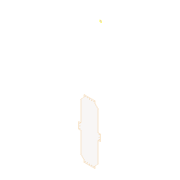
# Autodesk Inventor part: Test_Swerve_Center
Saved by Autodesk Inventor 2021 (Build 250183000, 183)
## iProperties
Created: 2023-03-29
Part Number: Test_Swerve_Center
Material: PMMA Plastic
Document SubType Name: Modeling
Designer: jackc
Density: 1.188 g/cm^3
Appearance: Polycarbonate - Smoked
Author: jackc
Autodesk Inventor part; units mm, degrees
ref_plane "YZ Plane" through (0, 0, 0) normal (1, 0, 0) x (0, 1, 0)
ref_plane "XZ Plane" through (0, 0, 0) normal (0, 1, 0) x (-1, 0, 0)
ref_plane "XY Plane" through (0, 0, 0) normal (0, 0, 1) x (1, 0, 0)
ref_plane "Work Plane3" through (0, 0, 0) normal (0, 0, 1) x (1, 0, 0)
sketch "Sketch1" plane through (0, 0, 0) normal (0, 0, 1) x (1, 0, 0)
  line L0 (-25.4, -893.191) -> (-25.4, -866.775) projected
  line L1 (-25.4, -893.191) -> (-23.241, -895.35) projected
  line L2 (-2.159, -895.35) -> (-23.241, -895.35) projected
  line L3 (-2.159, -895.35) -> (0, -893.191) projected
  line L4 (0, -866.775) -> (0, -893.191) projected
  arc A0 (3.175, -863.6) -> (0, -866.775) centre (3.175, -866.775) ccw projected
  line L5 (29.591, -863.6) -> (3.175, -863.6) projected
  line L6 (29.591, -863.6) -> (31.75, -861.441) projected
  line L7 (31.75, -840.359) -> (31.75, -861.441) projected
  line L8 (31.75, -840.359) -> (29.591, -838.2) projected
  line L9 (-54.991, -838.2) -> (29.591, -838.2) projected
  line L10 (-54.991, -838.2) -> (-57.15, -840.359) projected
  line L11 (-57.15, -861.441) -> (-57.15, -840.359) projected
  line L12 (-57.15, -861.441) -> (-54.991, -863.6) projected
  line L13 (-28.575, -863.6) -> (-54.991, -863.6) projected
  arc A1 (-25.4, -866.775) -> (-28.575, -863.6) centre (-28.575, -866.775) ccw projected
  circle A2 centre (12.7, -850.9) radius 2.0701 projected
  circle A3 centre (0, -850.9) radius 2.0701 projected
  circle A4 centre (-25.4, -850.9) radius 2.0701 projected
  circle A5 centre (-50.8, -850.9) radius 2.0701 projected
  circle A6 centre (-12.7, -876.3) radius 2.0701 projected
  circle A7 centre (-12.7, -863.6) radius 2.0701 projected
  circle A8 centre (-38.1, -850.9) radius 2.0701 projected
  circle A9 centre (-12.7, -850.9) radius 2.0701 projected
  circle A10 centre (-12.7, -889) radius 2.0701 projected
  circle A11 centre (25.4, -850.9) radius 2.0701 projected
  line L14 (-25.4, -863.6) -> (-25.4, -1498.6) construction
  line L15 (107.95, -863.6) -> (-361.95, -863.6) projected
  line L16 (-254, -893.191) -> (-254, -866.775) projected
  line L17 (-254, -893.191) -> (-251.841, -895.35) projected
  line L18 (-230.759, -895.35) -> (-251.841, -895.35) projected
  line L19 (-230.759, -895.35) -> (-228.6, -893.191) projected
  line L20 (-228.6, -866.775) -> (-228.6, -893.191) projected
  arc A12 (-225.425, -863.6) -> (-228.6, -866.775) centre (-225.425, -866.775) ccw projected
  line L21 (-199.009, -863.6) -> (-225.425, -863.6) projected
  line L22 (-199.009, -863.6) -> (-196.85, -861.441) projected
  line L23 (-196.85, -840.359) -> (-196.85, -861.441) projected
  line L24 (-196.85, -840.359) -> (-199.009, -838.2) projected
  line L25 (-283.591, -838.2) -> (-199.009, -838.2) projected
  line L26 (-283.591, -838.2) -> (-285.75, -840.359) projected
  line L27 (-285.75, -861.441) -> (-285.75, -840.359) projected
  line L28 (-285.75, -861.441) -> (-283.591, -863.6) projected
  line L29 (-257.175, -863.6) -> (-283.591, -863.6) projected
  arc A13 (-254, -866.775) -> (-257.175, -863.6) centre (-257.175, -866.775) ccw projected
  circle A14 centre (-215.9, -850.9) radius 2.0701 projected
  circle A15 centre (-228.6, -850.9) radius 2.0701 projected
  circle A16 centre (-254, -850.9) radius 2.0701 projected
  circle A17 centre (-279.4, -850.9) radius 2.0701 projected
  circle A18 centre (-241.3, -876.3) radius 2.0701 projected
  circle A19 centre (-241.3, -863.6) radius 2.0701 projected
  circle A20 centre (-266.7, -850.9) radius 2.0701 projected
  circle A21 centre (-241.3, -850.9) radius 2.0701 projected
  circle A22 centre (-241.3, -889) radius 2.0701 projected
  circle A23 centre (-203.2, -850.9) radius 2.0701 projected
  line L30 (-228.6, -863.6) -> (-228.6, -1498.6) projected
  line L31 (-361.95, -1498.6) -> (107.95, -1498.6) projected
  line L32 (0, -1469.009) -> (0, -1495.425) projected
  line L33 (0, -1469.009) -> (-2.159, -1466.85) projected
  line L34 (-23.241, -1466.85) -> (-2.159, -1466.85) projected
  line L35 (-23.241, -1466.85) -> (-25.4, -1469.009) projected
  line L36 (-25.4, -1495.425) -> (-25.4, -1469.009) projected
  arc A24 (-28.575, -1498.6) -> (-25.4, -1495.425) centre (-28.575, -1495.425) ccw projected
  line L37 (-54.991, -1498.6) -> (-28.575, -1498.6) projected
  line L38 (-54.991, -1498.6) -> (-57.15, -1500.759) projected
  line L39 (-57.15, -1521.841) -> (-57.15, -1500.759) projected
  line L40 (-57.15, -1521.841) -> (-54.991, -1524) projected
  line L41 (29.591, -1524) -> (-54.991, -1524) projected
  line L42 (29.591, -1524) -> (31.75, -1521.841) projected
  line L43 (31.75, -1500.759) -> (31.75, -1521.841) projected
  line L44 (31.75, -1500.759) -> (29.591, -1498.6) projected
  line L45 (3.175, -1498.6) -> (29.591, -1498.6) projected
  arc A25 (0, -1495.425) -> (3.175, -1498.6) centre (3.175, -1495.425) ccw projected
  circle A26 centre (-38.1, -1511.3) radius 2.0701 projected
  circle A27 centre (-25.4, -1511.3) radius 2.0701 projected
  circle A28 centre (0, -1511.3) radius 2.0701 projected
  circle A29 centre (25.4, -1511.3) radius 2.0701 projected
  circle A30 centre (-12.7, -1485.9) radius 2.0701 projected
  circle A31 centre (-12.7, -1498.6) radius 2.0701 projected
  circle A32 centre (12.7, -1511.3) radius 2.0701 projected
  circle A33 centre (-12.7, -1511.3) radius 2.0701 projected
  circle A34 centre (-12.7, -1473.2) radius 2.0701 projected
  circle A35 centre (-50.8, -1511.3) radius 2.0701 projected
  line L46 (-228.6, -1469.009) -> (-228.6, -1495.425) projected
  line L47 (-228.6, -1469.009) -> (-230.759, -1466.85) projected
  line L48 (-251.841, -1466.85) -> (-230.759, -1466.85) projected
  line L49 (-251.841, -1466.85) -> (-254, -1469.009) projected
  line L50 (-254, -1495.425) -> (-254, -1469.009) projected
  arc A36 (-257.175, -1498.6) -> (-254, -1495.425) centre (-257.175, -1495.425) ccw projected
  line L51 (-283.591, -1498.6) -> (-257.175, -1498.6) projected
  line L52 (-283.591, -1498.6) -> (-285.75, -1500.759) projected
  line L53 (-285.75, -1521.841) -> (-285.75, -1500.759) projected
  line L54 (-285.75, -1521.841) -> (-283.591, -1524) projected
  line L55 (-199.009, -1524) -> (-283.591, -1524) projected
  line L56 (-199.009, -1524) -> (-196.85, -1521.841) projected
  line L57 (-196.85, -1500.759) -> (-196.85, -1521.841) projected
  line L58 (-196.85, -1500.759) -> (-199.009, -1498.6) projected
  line L59 (-225.425, -1498.6) -> (-199.009, -1498.6) projected
  arc A37 (-228.6, -1495.425) -> (-225.425, -1498.6) centre (-225.425, -1495.425) ccw projected
  circle A38 centre (-266.7, -1511.3) radius 2.0701 projected
  circle A39 centre (-254, -1511.3) radius 2.0701 projected
  circle A40 centre (-228.6, -1511.3) radius 2.0701 projected
  circle A41 centre (-203.2, -1511.3) radius 2.0701 projected
  circle A42 centre (-241.3, -1485.9) radius 2.0701 projected
  circle A43 centre (-241.3, -1498.6) radius 2.0701 projected
  circle A44 centre (-215.9, -1511.3) radius 2.0701 projected
  circle A45 centre (-241.3, -1511.3) radius 2.0701 projected
  circle A46 centre (-241.3, -1473.2) radius 2.0701 projected
  circle A47 centre (-279.4, -1511.3) radius 2.0701 projected
  circle A48 centre (-76.2, -850.9) radius 2.0701 projected
  circle A49 centre (-101.6, -850.9) radius 2.0701 projected
  circle A50 centre (-127, -850.9) radius 2.0701 projected
  circle A51 centre (-152.4, -850.9) radius 2.0701 projected
  circle A52 centre (-177.8, -850.9) radius 2.0701 projected
  circle A53 centre (-76.2, -1511.3) radius 2.0701 projected
  circle A54 centre (-101.6, -1511.3) radius 2.0701 projected
  circle A55 centre (-127, -1511.3) radius 2.0701 projected
  circle A56 centre (-152.4, -1511.3) radius 2.0701 projected
  circle A57 centre (-177.8, -1511.3) radius 2.0701 projected
  circle A58 centre (-241.3, -1155.7) radius 2.0701 projected
  circle A59 centre (-241.3, -1181.1) radius 2.0701 projected
  circle A60 centre (-241.3, -1206.5) radius 2.0701 projected
  circle A61 centre (-12.7, -1181.1) radius 2.0701 projected
  circle A62 centre (-12.7, -1206.5) radius 2.0701 projected
  circle A63 centre (-12.7, -1155.7) radius 2.0701 projected
  line L60 (-63.5, -863.6) -> (-63.5, -838.2)
  line L61 (-63.5, -838.2) -> (-190.5, -838.2)
  line L62 (-190.5, -838.2) -> (-190.5, -863.6)
  line L63 (-25.4, -901.7) -> (-25.4, -1143)
  line L64 (0, -1143) -> (0, -1219.2)
  line L65 (0, -1219.2) -> (-25.4, -1219.2)
  line L66 (0, -1143) -> (-25.4, -1143)
  line L67 (-25.4, -1219.2) -> (-25.4, -1460.5)
  circle A64 centre (-12.7, -1155.7) radius 2.3813
  circle A65 centre (-12.7, -1181.1) radius 2.3812
  circle A66 centre (-12.7, -1206.5) radius 2.3813
  line L68 (-25.4, -901.7) -> (-63.5, -863.6)
  line L69 (-12.7, -1181.1) -> (-241.3, -1181.1)
  line L70 (-127, -850.9) -> (-127, -1511.3)
  line L71 (-228.6, -901.7) -> (-228.6, -1143)
  line L72 (-254, -1143) -> (-254, -1219.2)
  line L73 (-254, -1219.2) -> (-228.6, -1219.2)
  line L74 (-254, -1143) -> (-228.6, -1143)
  line L75 (-228.6, -1219.2) -> (-228.6, -1460.5)
  circle A67 centre (-241.3, -1155.7) radius 2.3813
  circle A68 centre (-241.3, -1181.1) radius 2.3812
  circle A69 centre (-241.3, -1206.5) radius 2.3813
  line L76 (-228.6, -901.7) -> (-190.5, -863.6)
  circle A70 centre (-177.8, -850.9) radius 2.3813
  circle A71 centre (-152.4, -850.9) radius 2.3813
  circle A72 centre (-127, -850.9) radius 2.3813
  circle A73 centre (-101.6, -850.9) radius 2.3813
  circle A74 centre (-76.2, -850.9) radius 2.3813
  line L77 (-63.5, -1498.6) -> (-63.5, -1524)
  line L78 (-63.5, -1524) -> (-190.5, -1524)
  line L79 (-190.5, -1524) -> (-190.5, -1498.6)
  line L80 (-25.4, -1460.5) -> (-63.5, -1498.6)
  line L81 (-228.6, -1460.5) -> (-190.5, -1498.6)
  circle A75 centre (-177.8, -1511.3) radius 2.3813
  circle A76 centre (-152.4, -1511.3) radius 2.3813
  circle A77 centre (-127, -1511.3) radius 2.3813
  circle A78 centre (-101.6, -1511.3) radius 2.3813
  circle A79 centre (-76.2, -1511.3) radius 2.3813
  point P0 (0, 0)
  dimension "d0" = 6.35
  dimension "d1" = 6.35
  dimension "d2" = 25.4
  dimension "d3" = 6.35
  dimension "d4" = 6.35
  dimension "d5" = 25.4
  dimension "d6" = 12.7
  dimension "d7" = 12.7
  dimension "d8" = 4.7625
  dimension "d9" = 4.7625
  dimension "d10" = 4.7625
  constraints: 44 end point, 17 symmetric about line, 16 centre point, 8 coincident, 5 equal radius, 3 perpendicular, 3 vertical, 1 horizontal, 1 parallel, 17 other
  measures "d0" distance between parallel lines of L60 L11
  measures "d1" distance between parallel lines of L23 L62
  measures "d2" distance of L61.end L62.end
  measures "d3" distance from line of L34 L67.end
  measures "d4" vertical distance of L63.start L1.end
  measures "d6" distance from line of A63.centre L66
  measures "d7" distance from line of L65 A62.centre
  measures "d8" diameter of A64
  measures "d9" diameter of A65
  measures "d10" diameter of A66
extrude "Extrusion1" add sketch "Sketch1" along normal blind 6.35 contours L68 L63 L66 L64 L65 L67 L80 L31 L70 L15 | L15 L62 L61 L60 | L70 L69 L30 L76 L15 | L70 L31 L81 L30 L69 | L30 L73 L72 L74 | L31 L77 L78 L79
equation "\"d9\" = d8"
equation "\"d10\" = d8"
body "Solid1"
